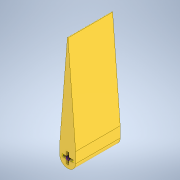
# Autodesk Inventor part: Bistable Flipper
Saved by Autodesk Inventor 2020 (Build 240168000, 168)
## iProperties
Created: 2019-11-08
Part Number: Bistable Flipper
Material: Generic
Document SubType Name: Modeling
Designer: camde
Density: 1 g/cm^3
Appearance: Glossy - Gold
Author: camde
Autodesk Inventor part; units mm, degrees
ref_plane "YZ Plane" through (0, 0, 0) normal (1, 0, 0) x (0, 1, 0)
ref_plane "XZ Plane" through (0, 0, 0) normal (0, 1, 0) x (-1, 0, 0)
ref_plane "XY Plane" through (0, 0, 0) normal (0, 0, 1) x (1, 0, 0)
sketch "Sketch1" plane through (0, 0, 0) normal (0, 0, 1) x (1, 0, 0)
  line L0 (-7.5832, 61.4886) -> (1.4084, 61.4886)
  line L1 (1.4084, 61.4886) -> (1.4084, -4.9324)
  line L2 (1.4084, -4.9324) -> (-7.5832, -4.9324)
  line L3 (-7.5832, -4.9324) -> (-7.5832, 61.4886)
  point P0 (0, 0)
  dimension "d0" = 8.9916
  dimension "d1" = 66.421
  constraints: 8 end point, 2 parallel, 1 horizontal, 1 perpendicular
  measures "d0" distance of L1.end L2.end
  measures "d1" distance of L0.end L1.end
extrude "Extrusion1" add sketch "Sketch1" along normal blind 25.4
sketch "Sketch2" plane through (0, 0, 25.4) normal (0, 0, 1) x (1, 0, 0)
  line L0 (-7.5832, -4.9324) -> (1.4084, -4.9324) projected
  line L1 (-3.0874, -4.9324) -> (-3.0874, 0.1476) construction
  circle A0 centre (-3.0874, 0.1476) radius 3.175 construction
  line L2 (-3.0874, 0.1476) -> (-3.7626, 3.25) construction
  line L3 (-3.0874, 0.1476) -> (-2.4123, 3.25) construction
  line L4 (-3.7626, 3.25) -> (-2.4123, 3.25)
  line L5 (-3.0874, 0.1476) -> (-6.1898, -0.5275) construction
  line L6 (-6.1898, -0.5275) -> (-6.1898, 0.8228)
  line L7 (-3.0874, 0.1476) -> (-2.4123, -2.9547) construction
  line L8 (-2.4123, -2.9547) -> (-3.7626, -2.9547)
  line L9 (-3.0874, 0.1476) -> (0.0149, 0.8228) construction
  line L10 (0.0149, 0.8228) -> (0.0149, -0.5275)
  line L11 (-3.7626, 3.25) -> (-3.7626, 0.8228)
  line L12 (-3.7626, -0.5275) -> (-3.7626, -2.9547)
  line L13 (-6.1898, -0.5275) -> (-3.7626, -0.5275)
  line L14 (-2.4123, -0.5275) -> (0.0149, -0.5275)
  line L15 (-2.4123, -2.9547) -> (-2.4123, -0.5275)
  line L16 (-2.4123, 0.8228) -> (-2.4123, 3.25)
  line L17 (-2.4123, 0.8228) -> (0.0149, 0.8228)
  line L18 (-6.1898, 0.8228) -> (-3.7626, 0.8228)
  point P0 (0, 0)
  dimension "d4" = 5.08
  dimension "d5" = 6.35
  dimension "d18" = 360
  constraints: 36 end point, 4 parallel, 3 horizontal, 3 vertical, 2 perpendicular, 2 point on circle, 1 centre point, 1 coincident, 1 midpoint, 21 other
  measures "d4" distance of L1.start L1.end
  measures "d5" diameter of A0
fillet "Fillet1" radius 4.4958 2 edges at (1.4084, -4.9324, 12.7) (-7.5832, -4.9324, 12.7)
chamfer "Chamfer1" distance 4.4958 distance2 55.88 1 edges at (-7.5832, 61.4886, 12.7) measured on face at (-1.5888, 61.4886, 8.4667)
chamfer "Chamfer2" distance 55.88 distance2 4.4958 1 edges at (1.4084, 61.4886, 12.7) measured on face at (1.4084, 20.2051, 8.4667)
sketch "Sketch3" plane through (0, 0, 25.4) normal (0, 0, 1) x (1, 0, 0)
  point P0 (0, 0)
fillet "Fillet2" radius 0.1588 2 edges at (-3.0873, 61.4886, 12.7) (-3.0874, 61.4886, 12.7)
extrude "Extrusion3" cut sketch "Sketch2" against normal blind 25.4
sketch "Sketch4" plane through (0, 0, 25.4) normal (0, 0, 1) x (1, 0, 0)
  line L0 (-6.1898, 0.8228) -> (-6.1898, -0.5275) projected
  line L1 (-6.1898, 0.1476) -> (-2.5733, 0.1476) construction
  circle A0 centre (-3.0874, 0.1476) radius 0.9548
  point P0 (0, 0)
  constraints: 2 end point, 1 centre point, 1 horizontal, 1 midpoint, 1 point on line
body "Solid1"
